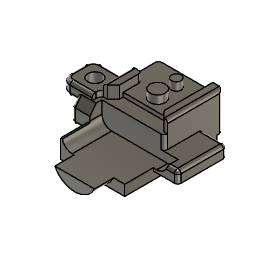
Sony PSP 2000 v5 v14 (Autodesk Fusion 360 design; units mm, degrees)
Autodesk Fusion 360 part; units mm, degrees
sketch "Boceto1" plane through (0, 0, 0) normal (0, 0, 1) x (1, 0, 0)
  line L0 (0, 12.0225) -> (7.85, 12.0225)
  line L1 (7.85, 12.0225) -> (7.85, 0.0225)
  line L2 (7.85, 0.0225) -> (0, 0.0225)
  line L3 (0, 0.0225) -> (0, 12.0225)
  dimension "d1" = 12
  dimension "d2" = 7.85
  constraint horizontal L0
  constraint vertical L1
  constraint horizontal L2
  constraint vertical L3
  measures "d1" distance of L0.end L1.end
  measures "d2" distance of L0.start L0.end
extrude "Extruir1" add sketch "Boceto1" along normal blind 5.51
sketch "Boceto2" plane through (0, 0, 0) normal (-1, 0, 0) x (0, -1, 0)
  line L0 (-12.0225, 0) -> (-0.0225, 0)
  line L1 (-0.0225, 0) -> (-0.0225, 5.51)
  line L2 (-0.0225, 5.51) -> (-12.0225, 5.51)
  line L3 (-12.0225, 5.51) -> (-12.0225, 0)
  line L4 (-12.0225, 0.85) -> (-11.3225, 0.85)
  line L5 (-11.3225, 0.85) -> (-11.3225, 0)
  line L6 (-8.0225, 4.71) -> (-4.1725, 4.71)
  line L7 (-4.1725, 4.71) -> (-4.1725, 3.1)
  line L8 (-4.1725, 3.1) -> (-8.0225, 3.1)
  line L9 (-8.0225, 3.1) -> (-8.0225, 4.71)
  line L10 (-7.7975, 3.1) -> (-7.7975, 1.15)
  line L11 (-7.7975, 1.15) -> (-8.7975, 1.15)
  line L12 (-8.7975, 1.15) -> (-8.7975, 2.988)
  line L13 (-8.0225, 4.01) -> (-8.7975, 2.988)
  line L14 (-3.3975, 2.988) -> (-3.3975, 1.15)
  line L15 (-3.3975, 1.15) -> (-4.3975, 1.15)
  line L16 (-4.3975, 1.15) -> (-4.3975, 3.1)
  line L17 (-4.1725, 4.01) -> (-3.3975, 2.988)
  dimension "d5" = 0.7
  dimension "d6" = 0.85
  dimension "d7" = 4
  dimension "d8" = 0.8
  dimension "d9" = 1.61
  dimension "d10" = 3.85
  dimension "d11" = 1
  dimension "d12" = 3.225
  dimension "d13" = 1.838
  dimension "d14" = 1.15
  dimension "d16" = 3.4
  dimension "d17" = 1
  dimension "d18" = 1.15
  dimension "d19" = 1.838
  dimension "d41" = 0.7
  dimension "d42" = 0.7
  constraint coincident L3 L4.start
  constraint perpendicular L3 L4
  constraint coincident L0 L5.end
  constraint perpendicular L0 L5
  constraint horizontal L6
  constraint vertical L7
  constraint horizontal L8
  constraint vertical L9
  constraint vertical L10
  constraint horizontal L11
  constraint vertical L12
  constraint vertical L14
  constraint horizontal L15
  constraint vertical L16
  constraint coincident L9 L13.start
  constraint coincident L8 L10.start
  constraint coincident L8 L16.end
  constraint coincident L7 L17.start
  measures "d5" distance of L4.start L4.end
  measures "d6" distance of L4.end L5.end
  measures "d7" horizontal distance of L2.end L6.start
  measures "d8" vertical distance of L2.end L6.start
  measures "d9" distance of L6.start L8.end
  measures "d10" distance of L6.start L6.end
  measures "d11" distance of L10.end L11.end
  measures "d12" horizontal distance of L0.start L11.end
  measures "d13" distance of L12.end L11.end
  measures "d14" vertical distance of L0.start L11.end
  measures "d16" horizontal distance of L10.end L15.end
  measures "d17" distance of L14.end L15.end
  measures "d18" vertical distance of L0.start L14.end
  measures "d19" distance of L14.start L14.end
  measures "d41" distance of L6.start L13.start
  measures "d42" distance of L6.end L17.start
extrude "Extruir2" cut sketch "Boceto2" against normal blind 7.85 contours L0 L3 L4 L5
extrude "Extruir3" add sketch "Boceto2" along normal blind 4 contours L6 L7 L8 L9
extrude "Extruir4" add sketch "Boceto2" along normal blind 2 contours L8 L9 L10 L11 L12 L13 | L7 L8 L14 L15 L16 L17
sketch "Boceto3" plane through (0, 0, 4.71) normal (0, 0, 1) x (-1, 0, 0)
  line L0 (0, -4.1725) -> (0, -8.0225)
  line L1 (0, -8.0225) -> (4, -8.0225)
  line L2 (4, -8.0225) -> (4, -4.1725)
  line L3 (4, -4.1725) -> (0, -4.1725)
  circle A0 centre (1.875, -6.0975) radius 0.875
  line L4 (0.3, -4.1725) -> (0.3, -5.2725)
  line L5 (0.3, -5.2725) -> (0, -5.2725)
  point P0 (1.875, -6.0975)
  dimension "d27" = 1.925
  dimension "d29" = 1.75
  dimension "d32" = 1.875
  dimension "d33" = 1.1
  dimension "d34" = 0.3
  constraint coincident P0 A0.centre
  constraint coincident L3 L4.start
  constraint perpendicular L3 L4
  constraint coincident L0 L5.end
  constraint perpendicular L0 L5
  measures "d27" vertical distance of L1.end P0
  measures "d29" diameter of A0
  measures "d32" horizontal distance of L0.end P0
  measures "d33" distance of L0.start L5.end
  measures "d34" distance of L0.start L4.start
extrude "Extruir5" cut sketch "Boceto3" against normal blind 1.61 contours A0
extrude "Extruir6" cut sketch "Boceto3" against normal blind 0.7 contours L0 L3 L4 L5
fillet "Empalme2" radius 1 2 edges at (-4, 4.1725, 3.905) (-4, 8.0225, 3.905)
fillet "Empalme1" radius 0.8 1 edges at (-0.3, 5.2725, 4.36)
sketch "Boceto4" plane through (0, 0.0225, 0) normal (0, -1, 0) x (1, 0, 0)
  line L0 (0, 0) -> (7.85, 0)
  line L1 (7.85, 0) -> (7.85, 5.51)
  line L2 (7.85, 5.51) -> (0, 5.51)
  line L3 (0, 5.51) -> (0, 0)
  line L4 (7.85, 1.295) -> (0.2, 1.295)
  arc A0 (1.6327, 1.295) -> (6.4973, 1.295) centre (4.065, 2.49) ccw
  line L5 (0.2, 1.295) -> (0.2, 4.01)
  line L6 (0.2, 4.01) -> (0, 4.01)
  line L7 (0.2, 2.295) -> (0, 2.295)
  point P0 (4.065, 2.49)
  dimension "d43" = 2.49
  dimension "d44" = 4.065
  dimension "d47" = 5.42
  dimension "d48" = 1.5
  dimension "d49" = 0.2
  dimension "d50" = 1.295
  dimension "d55" = 2.295
  constraint coincident L1 L4.start
  constraint perpendicular L3 L4
  constraint coincident P0 A0.centre
  constraint coincident L4 A0.start
  constraint coincident L4 A0.end
  constraint perpendicular L4 L5
  constraint coincident L3 L6.end
  constraint perpendicular L3 L6
  constraint coincident L5 L7.start
  constraint coincident L3 L7.end
  constraint perpendicular L3 L7
  measures "d43" vertical distance of L0.start A0.centre
  measures "d44" horizontal distance of L0.start A0.centre
  measures "d47" diameter of A0
  measures "d48" distance of L2.end L6.end
  measures "d49" distance of L5.end L6.end
  measures "d50" distance of L0.end L4.start
  measures "d55" distance of L0.start L7.end
extrude "Extruir7" add sketch "Boceto4" along normal blind 2.35 contours L0 L4 A0 | L0 A0
extrude "Extruir8" cut sketch "Boceto4" against normal blind 4.85 contours L1 L2 L3 L4 L5 L6
extrude "Extruir9" cut sketch "Boceto4" against normal blind 3.375 contours L3 L5 L6 L7
fillet "Empalme3" radius 1.2 1 edges at (0.2, 2.4475, 1.295)
extrude "Extruir10" cut 1 faces at (0, 3.6558, 3.6693) along direction (1, 0, 0) blind 0.2
sketch "Boceto5" plane through (7.85, 0, 0) normal (1, 0, 0) x (0, 1, 0)
  line L0 (4.8725, 5.51) -> (4.8725, 1.295)
  line L1 (4.8725, 1.295) -> (0.0225, 1.295)
  line L2 (0.0225, 1.295) -> (0.0225, 0)
  line L3 (0.0225, 0) -> (11.3225, 0)
  line L4 (11.3225, 0) -> (11.3225, 0.85)
  line L5 (11.3225, 0.85) -> (12.0225, 0.85)
  line L6 (12.0225, 0.85) -> (12.0225, 5.51)
  line L7 (12.0225, 5.51) -> (4.8725, 5.51)
  line L8 (9.5225, 2.35) -> (3.5225, 2.35)
  line L9 (3.5225, 2.35) -> (3.5225, 0.95)
  line L10 (3.5225, 0.95) -> (9.5225, 0.95)
  line L11 (9.5225, 0.95) -> (9.5225, 2.35)
  dimension "d62" = 0.95
  dimension "d63" = 1.4
  dimension "d64" = 6
  dimension "d65" = 2.5
  constraint horizontal L8
  constraint vertical L9
  constraint horizontal L10
  constraint vertical L11
  measures "d62" vertical distance of L3.end L10.end
  measures "d63" distance of L8.start L10.end
  measures "d64" distance of L9.end L10.end
  measures "d65" horizontal distance of L5.end L10.end
extrude "Extruir11" add sketch "Boceto5" along normal blind 3 contours L0 L1 L8 L9 L10 L11 | L0 L1 L8 L9
sketch "Boceto6" plane through (0, 3.5225, 0) normal (0, -1, 0) x (1, 0, 0)
  line L0 (7.85, 2.35) -> (7.85, 1.295)
  line L1 (7.85, 1.295) -> (7.85, 0.95)
  line L2 (7.85, 0.95) -> (10.85, 0.95)
  line L3 (10.85, 0.95) -> (10.85, 2.35)
  line L4 (10.85, 2.35) -> (7.85, 2.35)
  line L5 (7.85, 1.295) -> (9.55, 1.295)
  line L6 (9.55, 1.295) -> (9.55, 2.35)
  dimension "d68" = 1.7
  constraint coincident L0.end L1.start
  constraint perpendicular L0 L5
  constraint coincident L4 L6.end
  constraint perpendicular L4 L6
  measures "d68" distance of L0.start L6.end
extrude "Extruir12" cut sketch "Boceto6" against normal blind 1.35 contours L0 L4 L5 L6
fillet "Empalme4" radius 1.3 1 edges at (9.55, 4.1975, 1.295)
sketch "Boceto7" plane through (0, 0, 5.51) normal (0, 0, 1) x (-1, 0, 0)
  line L0 (0, -4.8725) -> (-7.85, -4.8725)
  line L1 (-7.85, -4.8725) -> (-7.85, -12.0225)
  line L2 (-7.85, -12.0225) -> (0, -12.0225)
  line L3 (0, -12.0225) -> (0, -4.8725)
  line L4 (0, -5.2725) -> (-0.45, -5.2725)
  line L5 (-0.45, -5.2725) -> (-1.2, -6.0225)
  line L6 (-1.2, -6.0225) -> (-1.2, -8.7725)
  line L7 (-1.2, -8.7725) -> (0, -8.7725)
  line L8 (-7.85, -5.2725) -> (-7.4, -5.2725)
  line L9 (-7.4, -5.2725) -> (-6.65, -6.0225)
  line L10 (-6.65, -6.0225) -> (-6.65, -12.0225)
  circle A0 centre (-3.925, -10.2625) radius 0.6
  circle A1 centre (-3.925, -7.9725) radius 0.95
  line L11 (-1.2, -6.4725) -> (-6.65, -6.4725)
  point P0 (-3.925, -10.2625)
  point P1 (-3.925, -7.9725)
  dimension "d73" = 1.2
  dimension "d74" = 1.2
  dimension "d75" = 0.45
  dimension "d76" = 0.45
  dimension "d77" = 0.75
  dimension "d78" = 6.75
  dimension "d79" = 0.4
  dimension "d80" = 0.4
  dimension "d81" = 0.75
  dimension "d82" = 1.76
  dimension "d83" = 4.05
  dimension "d84" = 3.925
  dimension "d85" = 3.925
  dimension "d86" = 1.2
  dimension "d87" = 1.9
  dimension "d88" = 1.6
  dimension "d95" = 3.25
  constraint coincident L3 L4.start
  constraint perpendicular L3 L4
  constraint parallel L3 L6
  constraint coincident L3 L7.end
  constraint perpendicular L3 L7
  constraint coincident L1 L8.start
  constraint perpendicular L1 L8
  constraint coincident L2 L10.end
  constraint perpendicular L2 L10
  constraint coincident P0 A0.centre
  constraint coincident P1 A1.centre
  constraint coincident L6 L11.start
  constraint coincident L10 L11.end
  constraint perpendicular L10 L11
  measures "d73" distance of L1.end L10.end
  measures "d74" distance of L6.end L7.end
  measures "d75" distance of L4.start L4.end
  measures "d76" distance of L8.start L8.end
  measures "d77" vertical distance of L8.start L9.end
  measures "d78" distance of L1.end L8.start
  measures "d79" distance of L0.end L8.start
  measures "d80" distance of L0.start L4.start
  measures "d81" vertical distance of L4.end L5.end
  measures "d82" distance of L2 P0
  measures "d83" distance of L2 P1
  measures "d84" horizontal distance of L2.end P0
  measures "d85" horizontal distance of L2.end P1
  measures "d86" diameter of A0
  measures "d87" diameter of A1
  measures "d88" vertical distance of L0.start L11.start
  measures "d95" distance of L2.end L7.end
extrude "Extruir13" cut sketch "Boceto7" against normal blind 1 contours L2 L3 L6 L7 L10 L11
extrude "Extruir14" cut sketch "Boceto7" against normal blind 1.5 contours L0 L1 L3 L4 L5 L6 L8 L9 L10 L11
fillet "Empalme5" radius 0.4 1 edges at (1.2, 8.7725, 5.01)
fillet "Empalme6" radius 0.4 30 edges at (10.85, 6.5225, 2.35) (10.85, 3.5225, 1.65) (10.85, 9.5225, 1.65) (9.35, 9.5225, 2.35) (7.85, 12.0225, 3.18) (7.85, 8.6475, 5.51) (0, 12.0225, 2.68) (0, 7.0225, 5.51) (-1.5, 8.0225, 4.71) (-3.7071, 7.7296, 4.71) (-4, 6.0975, 4.71) (-3.7071, 4.4654, 4.71) (-1.65, 4.1725, 4.71) (-2.5, 4.1725, 3.1) (-3.7071, 4.4654, 3.1) (-4, 6.0975, 3.1) (-3.7071, 7.7296, 3.1) (-2.5, 8.0225, 3.1) (-2, 8.7975, 2.069) (-2, 3.3975, 2.069) (10.2, 3.5225, 2.35) (-2, 8.41, 3.499) (-2, 3.785, 3.499) (-1, 3.3975, 1.15) (-1, 4.3975, 1.15) (-1, 7.7975, 1.15) (-1, 8.7975, 1.15) (-2, 8.2975, 1.15) (-2, 3.8975, 1.15) (7.85, 4.8725, 3.18)
other "Elemento de malla base1"
equation "d17 = d11"
equation "d18 = d14"
equation "d19 = d13"
equation "d21 = -d2"
equation "d27 = d10 / 2"
equation "d30 = -d9"
equation "d35 = -d41"
equation "d42 = d41"
equation "d43 = 2.23 mm + 0.26 mm"
equation "d48 = d8 + d41"
equation "d60 = -d49"
equation "d73 = d74"
equation "d76 = d75"
equation "d77 = d81"
equation "d84 = d85"
